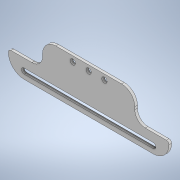
# Autodesk Inventor part: NEW Бампер
Saved by Autodesk Inventor 2021 (Build 250183000, 183)
## iProperties
Created: 2022-07-08
Part Number: NEW Бампер
Material: Типовые
Document SubType Name: Modeling
Designer: zvi20
Density: 1 g/cm^3
Appearance: По умолчанию
Author: zvi20
Autodesk Inventor part; units mm, degrees
ref_plane "YZ Plane" through (0, 0, 0) normal (1, 0, 0) x (0, 1, 0)
ref_plane "XZ Plane" through (0, 0, 0) normal (0, 1, 0) x (-1, 0, 0)
ref_plane "XY Plane" through (0, 0, 0) normal (0, 0, 1) x (1, 0, 0)
sketch "Эскиз1" plane through (0, 0, 0) normal (0, 0, 1) x (1, 0, 0)
  line L0 (1380.315, -1246.7097) -> (1380.315, -1245.7097)
  line L1 (1390.315, -1235.7097) -> (1440.315, -1235.7097)
  line L2 (1450.315, -1245.7097) -> (1450.315, -1246.7097)
  arc A0 (1390.315, -1235.7097) -> (1380.315, -1245.7097) centre (1390.315, -1245.7097) ccw
  arc A1 (1450.315, -1245.7097) -> (1440.315, -1235.7097) centre (1440.315, -1245.7097) ccw
  line L3 (1380.315, -1246.7097) -> (1380.315, -1247.7097)
  line L4 (1372.315, -1255.7097) -> (1357.315, -1255.7097)
  line L5 (1473.3109, -1255.7097) -> (1458.315, -1255.7097)
  line L6 (1450.315, -1247.7097) -> (1450.315, -1246.7097)
  arc A2 (1372.315, -1255.7097) -> (1380.315, -1247.7097) centre (1372.315, -1247.7097) ccw
  arc A3 (1450.315, -1247.7097) -> (1458.315, -1255.7097) centre (1458.315, -1247.7097) ccw
  circle A4 centre (1415.315, -1239.7097) radius 2
  line L7 (1357.315, -1255.7097) -> (1356.315, -1255.7097)
  arc A5 (1356.315, -1255.7097) -> (1354.315, -1257.7097) centre (1356.315, -1257.7097) ccw
  line L8 (1473.3109, -1255.7097) -> (1474.3062, -1255.7097)
  arc A6 (1476.3062, -1257.7097) -> (1474.3062, -1255.7097) centre (1474.3062, -1257.7097) ccw
  circle A7 centre (1427.315, -1239.7097) radius 2
  arc A8 (1366.3109, -1262.2097) -> (1366.3109, -1266.2097) centre (1366.3109, -1264.2097) ccw
  arc A9 (1464.3109, -1266.2097) -> (1464.3109, -1262.2097) centre (1464.3109, -1264.2097) ccw
  line L9 (1366.3109, -1262.2097) -> (1464.3109, -1262.2097)
  line L10 (1464.3109, -1266.2097) -> (1366.3109, -1266.2097)
  line L11 (1366.315, -1269.7097) -> (1464.3062, -1269.7097)
  line L12 (1476.3062, -1257.7097) -> (1476.3062, -1257.7097)
  line L13 (1354.315, -1257.7097) -> (1354.315, -1257.7097)
  arc A10 (1354.315, -1257.7097) -> (1366.315, -1269.7097) centre (1366.315, -1257.7097) ccw
  arc A11 (1464.3062, -1269.7097) -> (1476.3062, -1257.7097) centre (1464.3062, -1257.7097) ccw
  circle A12 centre (1403.315, -1239.7097) radius 2
  point P0 (0, 0)
  point P1 (1450.315, -1235.7097)
  point P2 (1380.315, -1255.7097)
  point P3 (1354.315, -1255.7097)
  point P4 (1476.3109, -1270.2097)
  constraints: 28 end point, 20 point on circle, 16 tangent, 13 centre point, 6 point on line, 5 perpendicular, 3 vertical, 2 equal radius, 2 horizontal
extrude "Выдавливание3" add sketch "Эскиз1" along normal blind 2
